Autodesk Inventor part; units mm, degrees
(part 2 of 2)
  line L427 (263.1, -57.6) -> (263.1, -56.8)
  line L428 (263.1, -57.6) -> (263.1, -58.4)
  arc A171 (259.4858, -61.6) -> (260.1929, -61.3071) centre (259.4858, -60.6) ccw
  line L429 (260.1929, -61.3071) -> (263.1, -58.4)
  line L430 (-262.2, 25.9) -> (-263.8, 25.9)
  line L431 (-263.8, 25.9) -> (-267, 22.7)
  line L432 (-267, 22.7) -> (-271.0621, -34.3)
  line L433 (-263.0621, -34.3) -> (-259, 22.7)
  line L434 (-259, 22.7) -> (-262.2, 25.9)
  line L435 (-271.0621, -34.3) -> (-267.8621, -37.5)
  line L436 (-267.8621, -37.5) -> (-266.2621, -37.5)
  line L437 (-266.2621, -37.5) -> (-263.0621, -34.3)
  line L438 (-217, 20.5) -> (-219.9071, 17.5929)
  line L439 (-220.2, 16.8858) -> (-220.2, -0.3)
  line L440 (-237.3858, -0.3) -> (-220.2, -0.3)
  line L441 (-238.0929, -0.5929) -> (-241, -3.5)
  line L442 (-241, -3.5) -> (-241, -5.1)
  line L443 (-237.3858, -8.3) -> (-220.2, -8.3)
  line L444 (-220.2, -8.3) -> (-220.2, -25.4858)
  line L445 (-217, -29.1) -> (-215.4, -29.1)
  line L446 (-215.4, -29.1) -> (-212.4929, -26.1929)
  line L447 (-212.2, -25.4858) -> (-212.2, -8.3)
  line L448 (-195.0142, -0.3) -> (-212.2, -0.3)
  line L449 (-195.0142, -8.3) -> (-212.2, -8.3)
  line L450 (-194.3071, -0.5929) -> (-191.4, -3.5)
  line L451 (-191.4, -3.5) -> (-191.4, -5.1)
  line L452 (-238.0929, -8.0071) -> (-241, -5.1)
  line L453 (-219.9071, -26.1929) -> (-217, -29.1)
  line L454 (-194.3071, -8.0071) -> (-191.4, -5.1)
  line L455 (-212.2, -0.3) -> (-212.2, 16.8858)
  line L456 (-212.4929, 17.5929) -> (-215.4, 20.5)
  line L457 (-215.4, 20.5) -> (-217, 20.5)
  arc A172 (-219.9071, 17.5929) -> (-220.2, 16.8858) centre (-219.2, 16.8858) ccw
  arc A173 (-212.2, 16.8858) -> (-212.4929, 17.5929) centre (-213.2, 16.8858) ccw
  arc A174 (-194.3071, -0.5929) -> (-195.0142, -0.3) centre (-195.0142, -1.3) ccw
  arc A175 (-195.0142, -8.3) -> (-194.3071, -8.0071) centre (-195.0142, -7.3) ccw
  arc A176 (-220.2, -25.4858) -> (-219.9071, -26.1929) centre (-219.2, -25.4858) ccw
  arc A177 (-212.4929, -26.1929) -> (-212.2, -25.4858) centre (-213.2, -25.4858) ccw
  arc A178 (-238.0929, -8.0071) -> (-237.3858, -8.3) centre (-237.3858, -7.3) ccw
  arc A179 (-237.3858, -0.3) -> (-238.0929, -0.5929) centre (-237.3858, -1.3) ccw
  line L458 (-34.2, 15) -> (-32.2, 15)
  line L459 (-32.2, 15) -> (-29, 11.8)
  line L460 (-29, 11.8) -> (-29, 9.8)
  line L461 (-29, 9.8) -> (-32.2, 6.6)
  line L462 (-32.2, 6.6) -> (-34.2, 6.6)
  line L463 (-34.2, 6.6) -> (-37.4, 9.8)
  line L464 (-37.4, 9.8) -> (-37.4, 11.8)
  line L465 (-37.4, 11.8) -> (-34.2, 15)
  line L466 (-34.2, -14.4) -> (-32.2, -14.4)
  line L467 (-32.2, -14.4) -> (-29, -17.6)
  line L468 (-29, -17.6) -> (-29, -19.6)
  line L469 (-29, -19.6) -> (-32.2, -22.8)
  line L470 (-32.2, -22.8) -> (-34.2, -22.8)
  line L471 (-34.2, -22.8) -> (-37.4, -19.6)
  line L472 (-37.4, -19.6) -> (-37.4, -17.6)
  line L473 (-37.4, -17.6) -> (-34.2, -14.4)
  line L474 (121.9, 15) -> (123.9, 15)
  line L475 (123.9, 15) -> (127.1, 11.8)
  line L476 (127.1, 11.8) -> (127.1, 9.8)
  line L477 (127.1, 9.8) -> (123.9, 6.6)
  line L478 (123.9, 6.6) -> (121.9, 6.6)
  line L479 (121.9, 6.6) -> (118.7, 9.8)
  line L480 (118.7, 9.8) -> (118.7, 11.8)
  line L481 (118.7, 11.8) -> (121.9, 15)
  line L482 (121.9, -14.4) -> (123.9, -14.4)
  line L483 (123.9, -14.4) -> (127.1, -17.6)
  line L484 (127.1, -17.6) -> (127.1, -19.6)
  line L485 (127.1, -19.6) -> (123.9, -22.8)
  line L486 (123.9, -22.8) -> (121.9, -22.8)
  line L487 (121.9, -22.8) -> (118.7, -19.6)
  line L488 (118.7, -19.6) -> (118.7, -17.6)
  line L489 (118.7, -17.6) -> (121.9, -14.4)
  point P0 (-22.4267, -1.12)
  dimension "d244" = 0
  dimension "d246" = 0
  dimension "d247" = 0
  dimension "d248" = 0
  dimension "d249" = 10
  dimension "d250" = 7.5
  dimension "d251" = 25
  dimension "d252" = 7.5
  dimension "d253" = 25
  dimension "d308" = 1.1
  dimension "d309" = 21
  dimension "d310" = 21
  dimension "d324" = 21
  dimension "d325" = 0
  dimension "d326" = 21
  dimension "d327" = 21
  dimension "d328" = 0
  dimension "d329" = 21
  dimension "d330" = 39
  dimension "d334" = 0
  dimension "d335" = 18
  dimension "d336" = 23
  dimension "d339" = 11.5
  dimension "d341" = 11.5
sketch "Clock Front Face Outline" plane through (0, 0, 0) normal (0, 0, 1) x (1, 0, 0)
  line L0 (-99.6752, 68) -> (99.6752, 68)
  line L1 (300, 16.6643) -> (300, -28.3498)
  line L2 (-300, -28.3498) -> (-300, 16.6643)
  arc A0 (261.5609, 58.5131) -> (100.3256, 67.9894) centre (0, -3015.4231) ccw
  arc A1 (-100.3256, 67.9894) -> (-261.5609, 58.5131) centre (0, -3015.4231) ccw
  line L3 (-159.5034, -75) -> (159.5034, -75)
  arc A2 (-263.2612, -68.2167) -> (-160.4975, -74.9753) centre (0, 3150) ccw
  arc A3 (160.4975, -74.9753) -> (263.2612, -68.2167) centre (0, 3150) ccw
  arc A4 (300, 16.6643) -> (261.5609, 58.5131) centre (258, 16.6643) ccw
  arc A5 (263.2612, -68.2167) -> (300, -28.3498) centre (260, -28.3498) ccw
  arc A6 (-300, -28.3498) -> (-263.2612, -68.2167) centre (-260, -28.3498) ccw
  arc A7 (-261.5609, 58.5131) -> (-300, 16.6643) centre (-258, 16.6643) ccw
  arc A8 (-99.6752, 68) -> (-100.3256, 67.9894) centre (-99.6752, 48) ccw
  arc A9 (100.3256, 67.9894) -> (99.6752, 68) centre (99.6752, 48) ccw
  arc A10 (159.5034, -75) -> (160.4975, -74.9753) centre (159.5034, -55) ccw
  arc A11 (-160.4975, -74.9753) -> (-159.5034, -75) centre (-159.5034, -55) ccw
  point P0 (0, -2.2582)
  point P1 (-100, 68)
  point P2 (100, 68)
  point P3 (-300, 55)
  point P4 (300, 55)
  point P5 (-300, -65)
  point P6 (300, -65)
  point P7 (-160, -75)
  point P8 (160, -75)
  dimension "d0" = 600
  dimension "d4" = 120
  dimension "d5" = 120
  dimension "d12" = 140
  dimension "d13" = 140
  dimension "d14" = 200
  dimension "d15" = 200
  dimension "d16" = 200
  dimension "d17" = 320
  dimension "d18" = 143
  dimension "d19" = 10
  dimension "d20" = 10
  dimension "d21" = 13
  dimension "d22" = 13
  dimension "d24" = 42
  dimension "d25" = 40
  dimension "d26" = 40
  dimension "d27" = 42
  dimension "d28" = 20
  measures "d0" distance between parallel lines of L1 L2
  measures "d4" distance of point (-300, 55) point (-300, -65)
  measures "d5" distance of point (300, 55) point (300, -65)
  measures "d12" horizontal distance of point (-300, -65) point (-160, -75)
  measures "d13" horizontal distance of point (300, -65) point (160, -75)
  measures "d14" horizontal distance of point (-300, 55) point (-100, 68)
  measures "d15" horizontal distance of point (300, 55) point (100, 68)
  measures "d16" distance of point (100, 68) point (-100, 68)
  measures "d17" distance of point (160, -75) point (-160, -75)
  measures "d18" distance from line of L3 point (-100, 68)
  measures "d19" vertical distance of point (-300, -65) point (-160, -75)
  measures "d20" vertical distance of point (300, -65) point (160, -75)
  measures "d21" vertical distance of point (100, 68) point (300, 55)
  measures "d22" vertical distance of point (-100, 68) point (-300, 55)
  measures "d24" radius of A4
  measures "d25" radius of A5
  measures "d26" radius of A6
  measures "d27" radius of A7
  measures "d28" radius of A8
sketch "Sketch1" plane through (0, 0, 0) normal (0, 0, 1) x (1, 0, 0)
  line L0 (-99.6752, 68) -> (99.6752, 68)
  line L1 (300, 16.6643) -> (300, -28.3498)
  line L2 (-300, -28.3498) -> (-300, 16.6643)
  arc A0 (261.5609, 58.5131) -> (100.3256, 67.9894) centre (0, -3015.4231) ccw
  arc A1 (-100.3256, 67.9894) -> (-261.5609, 58.5131) centre (0, -3015.4231) ccw
  line L3 (-159.5034, -75) -> (159.5034, -75)
  arc A2 (-263.2612, -68.2167) -> (-160.4975, -74.9753) centre (0, 3150) ccw
  arc A3 (160.4975, -74.9753) -> (263.2612, -68.2167) centre (0, 3150) ccw
  arc A4 (300, 16.6643) -> (261.5609, 58.5131) centre (258, 16.6643) ccw
  arc A5 (263.2612, -68.2167) -> (300, -28.3498) centre (260, -28.3498) ccw
  arc A6 (-300, -28.3498) -> (-263.2612, -68.2167) centre (-260, -28.3498) ccw
  arc A7 (-261.5609, 58.5131) -> (-300, 16.6643) centre (-258, 16.6643) ccw
  arc A8 (-99.6752, 68) -> (-100.3256, 67.9894) centre (-99.6752, 48) ccw
  arc A9 (100.3256, 67.9894) -> (99.6752, 68) centre (99.6752, 48) ccw
  arc A10 (159.5034, -75) -> (160.4975, -74.9753) centre (159.5034, -55) ccw
  arc A11 (-160.4975, -74.9753) -> (-159.5034, -75) centre (-159.5034, -55) ccw
  point P0 (0, 0)
  dimension "d2" = 300
  dimension "d23" = 75
extrude "Extrusion1" add sketch "Sketch1" along normal blind 3
sketch "Sketch4" plane through (0, 0, 3) normal (0, 0, 1) x (1, 0, 0)
  line L0 (-300, 16.6643) -> (-300, -28.3498) projected
  line L1 (99.6752, 68) -> (-99.6752, 68) projected
  line L2 (-159.5034, -75) -> (159.5034, -75) projected
  line L3 (300, -28.3498) -> (300, 16.6643) projected
  arc A0 (144.2071, 46.2929) -> (144.9142, 46) centre (144.9142, 47) ccw
  arc A1 (144.9142, 54) -> (144.2071, 53.7071) centre (144.9142, 53) ccw
  line L4 (144.2071, 46.2929) -> (141.3, 49.2)
  line L5 (144.2071, 53.7071) -> (141.3, 50.8)
  line L6 (141.3, 50) -> (141.3, 49.2)
  line L7 (141.3, 50) -> (141.3, 50.8)
  line L8 (144.9142, 54) -> (187.6858, 54)
  line L9 (187.6858, 46) -> (144.9142, 46)
  arc A2 (188.3929, 53.7071) -> (187.6858, 54) centre (187.6858, 53) ccw
  line L10 (188.3929, 53.7071) -> (191.3, 50.8)
  line L11 (191.3, 50) -> (191.3, 50.8)
  line L12 (191.3, 50) -> (191.3, 49.2)
  arc A3 (187.6858, 46) -> (188.3929, 46.2929) centre (187.6858, 47) ccw
  line L13 (188.3929, 46.2929) -> (191.3, 49.2)
  arc A4 (144.2071, -7.5071) -> (144.9142, -7.8) centre (144.9142, -6.8) ccw
  arc A5 (144.9142, 0.2) -> (144.2071, -0.0929) centre (144.9142, -0.8) ccw
  line L14 (144.2071, -7.5071) -> (141.3, -4.6)
  line L15 (144.2071, -0.0929) -> (141.3, -3)
  line L16 (141.3, -3.8) -> (141.3, -4.6)
  line L17 (141.3, -3.8) -> (141.3, -3)
  line L18 (144.9142, 0.2) -> (187.6858, 0.2)
  line L19 (187.6858, -7.8) -> (144.9142, -7.8)
  arc A6 (188.3929, -0.0929) -> (187.6858, 0.2) centre (187.6858, -0.8) ccw
  line L20 (188.3929, -0.0929) -> (191.3, -3)
  line L21 (191.3, -3.8) -> (191.3, -3)
  line L22 (191.3, -3.8) -> (191.3, -4.6)
  arc A7 (187.6858, -7.8) -> (188.3929, -7.5071) centre (187.6858, -6.8) ccw
  line L23 (188.3929, -7.5071) -> (191.3, -4.6)
  arc A8 (143.1071, 1.0071) -> (143.4, 1.7142) centre (142.4, 1.7142) ccw
  arc A9 (135.4, 1.7142) -> (135.6929, 1.0071) centre (136.4, 1.7142) ccw
  line L24 (143.1071, 1.0071) -> (140.2, -1.9)
  line L25 (135.6929, 1.0071) -> (138.6, -1.9)
  line L26 (139.4, -1.9) -> (140.2, -1.9)
  line L27 (139.4, -1.9) -> (138.6, -1.9)
  line L28 (135.4, 1.7142) -> (135.4, 44.4858)
  line L29 (143.4, 44.4858) -> (143.4, 1.7142)
  arc A10 (135.6929, 45.1929) -> (135.4, 44.4858) centre (136.4, 44.4858) ccw
  line L30 (135.6929, 45.1929) -> (138.6, 48.1)
  line L31 (139.4, 48.1) -> (138.6, 48.1)
  line L32 (139.4, 48.1) -> (140.2, 48.1)
  arc A11 (143.4, 44.4858) -> (143.1071, 45.1929) centre (142.4, 44.4858) ccw
  line L33 (143.1071, 45.1929) -> (140.2, 48.1)
  arc A12 (143.1071, -52.7929) -> (143.4, -52.0858) centre (142.4, -52.0858) ccw
  arc A13 (135.4, -52.0858) -> (135.6929, -52.7929) centre (136.4, -52.0858) ccw
  line L34 (143.1071, -52.7929) -> (140.2, -55.7)
  line L35 (135.6929, -52.7929) -> (138.6, -55.7)
  line L36 (139.4, -55.7) -> (140.2, -55.7)
  line L37 (139.4, -55.7) -> (138.6, -55.7)
  line L38 (135.4, -52.0858) -> (135.4, -9.3142)
  line L39 (143.4, -9.3142) -> (143.4, -52.0858)
  arc A14 (135.6929, -8.6071) -> (135.4, -9.3142) centre (136.4, -9.3142) ccw
  line L40 (135.6929, -8.6071) -> (138.6, -5.7)
  line L41 (139.4, -5.7) -> (138.6, -5.7)
  line L42 (139.4, -5.7) -> (140.2, -5.7)
  arc A15 (143.4, -9.3142) -> (143.1071, -8.6071) centre (142.4, -9.3142) ccw
  line L43 (143.1071, -8.6071) -> (140.2, -5.7)
  arc A16 (196.9071, 1.0071) -> (197.2, 1.7142) centre (196.2, 1.7142) ccw
  arc A17 (189.2, 1.7142) -> (189.4929, 1.0071) centre (190.2, 1.7142) ccw
  line L44 (196.9071, 1.0071) -> (194, -1.9)
  line L45 (189.4929, 1.0071) -> (192.4, -1.9)
  line L46 (193.2, -1.9) -> (194, -1.9)
  line L47 (193.2, -1.9) -> (192.4, -1.9)
  line L48 (189.2, 1.7142) -> (189.2, 44.4858)
  line L49 (197.2, 44.4858) -> (197.2, 1.7142)
  arc A18 (189.4929, 45.1929) -> (189.2, 44.4858) centre (190.2, 44.4858) ccw
  line L50 (189.4929, 45.1929) -> (192.4, 48.1)
  line L51 (193.2, 48.1) -> (192.4, 48.1)
  line L52 (193.2, 48.1) -> (194, 48.1)
  arc A19 (197.2, 44.4858) -> (196.9071, 45.1929) centre (196.2, 44.4858) ccw
  line L53 (196.9071, 45.1929) -> (194, 48.1)
  arc A20 (196.9071, -52.7929) -> (197.2, -52.0858) centre (196.2, -52.0858) ccw
  arc A21 (189.2, -52.0858) -> (189.4929, -52.7929) centre (190.2, -52.0858) ccw
  line L54 (196.9071, -52.7929) -> (194, -55.7)
  line L55 (189.4929, -52.7929) -> (192.4, -55.7)
  line L56 (193.2, -55.7) -> (194, -55.7)
  line L57 (193.2, -55.7) -> (192.4, -55.7)
  line L58 (189.2, -52.0858) -> (189.2, -9.3142)
  line L59 (197.2, -9.3142) -> (197.2, -52.0858)
  arc A22 (189.4929, -8.6071) -> (189.2, -9.3142) centre (190.2, -9.3142) ccw
  line L60 (189.4929, -8.6071) -> (192.4, -5.7)
  line L61 (193.2, -5.7) -> (192.4, -5.7)
  line L62 (193.2, -5.7) -> (194, -5.7)
  arc A23 (197.2, -9.3142) -> (196.9071, -8.6071) centre (196.2, -9.3142) ccw
  line L63 (196.9071, -8.6071) -> (194, -5.7)
  arc A24 (144.2071, -61.3071) -> (144.9142, -61.6) centre (144.9142, -60.6) ccw
  arc A25 (144.9142, -53.6) -> (144.2071, -53.8929) centre (144.9142, -54.6) ccw
  line L64 (144.2071, -61.3071) -> (141.3, -58.4)
  line L65 (144.2071, -53.8929) -> (141.3, -56.8)
  line L66 (141.3, -57.6) -> (141.3, -58.4)
  line L67 (141.3, -57.6) -> (141.3, -56.8)
  line L68 (144.9142, -53.6) -> (187.6858, -53.6)
  line L69 (187.6858, -61.6) -> (144.9142, -61.6)
  arc A26 (188.3929, -53.8929) -> (187.6858, -53.6) centre (187.6858, -54.6) ccw
  line L70 (188.3929, -53.8929) -> (191.3, -56.8)
  line L71 (191.3, -57.6) -> (191.3, -56.8)
  line L72 (191.3, -57.6) -> (191.3, -58.4)
  arc A27 (187.6858, -61.6) -> (188.3929, -61.3071) centre (187.6858, -60.6) ccw
  line L73 (188.3929, -61.3071) -> (191.3, -58.4)
  arc A28 (57.4071, 46.2929) -> (58.1142, 46) centre (58.1142, 47) ccw
  arc A29 (58.1142, 54) -> (57.4071, 53.7071) centre (58.1142, 53) ccw
  line L74 (57.4071, 46.2929) -> (54.5, 49.2)
  line L75 (57.4071, 53.7071) -> (54.5, 50.8)
  line L76 (54.5, 50) -> (54.5, 49.2)
  line L77 (54.5, 50) -> (54.5, 50.8)
  line L78 (58.1142, 54) -> (100.8858, 54)
  line L79 (100.8858, 46) -> (58.1142, 46)
  arc A30 (101.5929, 53.7071) -> (100.8858, 54) centre (100.8858, 53) ccw
  line L80 (101.5929, 53.7071) -> (104.5, 50.8)
  line L81 (104.5, 50) -> (104.5, 50.8)
  line L82 (104.5, 50) -> (104.5, 49.2)
  arc A31 (100.8858, 46) -> (101.5929, 46.2929) centre (100.8858, 47) ccw
  line L83 (101.5929, 46.2929) -> (104.5, 49.2)
  arc A32 (57.4071, -7.5071) -> (58.1142, -7.8) centre (58.1142, -6.8) ccw
  arc A33 (58.1142, 0.2) -> (57.4071, -0.0929) centre (58.1142, -0.8) ccw
  line L84 (57.4071, -7.5071) -> (54.5, -4.6)
  line L85 (57.4071, -0.0929) -> (54.5, -3)
  line L86 (54.5, -3.8) -> (54.5, -4.6)
  line L87 (54.5, -3.8) -> (54.5, -3)
  line L88 (58.1142, 0.2) -> (100.8858, 0.2)
  line L89 (100.8858, -7.8) -> (58.1142, -7.8)
  arc A34 (101.5929, -0.0929) -> (100.8858, 0.2) centre (100.8858, -0.8) ccw
  line L90 (101.5929, -0.0929) -> (104.5, -3)
  line L91 (104.5, -3.8) -> (104.5, -3)
  line L92 (104.5, -3.8) -> (104.5, -4.6)
  arc A35 (100.8858, -7.8) -> (101.5929, -7.5071) centre (100.8858, -6.8) ccw
  line L93 (101.5929, -7.5071) -> (104.5, -4.6)
  arc A36 (56.3071, 1.0071) -> (56.6, 1.7142) centre (55.6, 1.7142) ccw
  arc A37 (48.6, 1.7142) -> (48.8929, 1.0071) centre (49.6, 1.7142) ccw
  line L94 (56.3071, 1.0071) -> (53.4, -1.9)
  line L95 (48.8929, 1.0071) -> (51.8, -1.9)
  line L96 (52.6, -1.9) -> (53.4, -1.9)
  line L97 (52.6, -1.9) -> (51.8, -1.9)
  line L98 (48.6, 1.7142) -> (48.6, 44.4858)
  line L99 (56.6, 44.4858) -> (56.6, 1.7142)
  arc A38 (48.8929, 45.1929) -> (48.6, 44.4858) centre (49.6, 44.4858) ccw
  line L100 (48.8929, 45.1929) -> (51.8, 48.1)
  line L101 (52.6, 48.1) -> (51.8, 48.1)
  line L102 (52.6, 48.1) -> (53.4, 48.1)
  arc A39 (56.6, 44.4858) -> (56.3071, 45.1929) centre (55.6, 44.4858) ccw
  line L103 (56.3071, 45.1929) -> (53.4, 48.1)
  arc A40 (56.3071, -52.7929) -> (56.6, -52.0858) centre (55.6, -52.0858) ccw
  arc A41 (48.6, -52.0858) -> (48.8929, -52.7929) centre (49.6, -52.0858) ccw
  line L104 (56.3071, -52.7929) -> (53.4, -55.7)
  line L105 (48.8929, -52.7929) -> (51.8, -55.7)
  line L106 (52.6, -55.7) -> (53.4, -55.7)
  line L107 (52.6, -55.7) -> (51.8, -55.7)
  line L108 (48.6, -52.0858) -> (48.6, -9.3142)
  line L109 (56.6, -9.3142) -> (56.6, -52.0858)
  arc A42 (48.8929, -8.6071) -> (48.6, -9.3142) centre (49.6, -9.3142) ccw
  line L110 (48.8929, -8.6071) -> (51.8, -5.7)
  line L111 (52.6, -5.7) -> (51.8, -5.7)
  line L112 (52.6, -5.7) -> (53.4, -5.7)
  arc A43 (56.6, -9.3142) -> (56.3071, -8.6071) centre (55.6, -9.3142) ccw
  line L113 (56.3071, -8.6071) -> (53.4, -5.7)
  arc A44 (110.1071, 1.0071) -> (110.4, 1.7142) centre (109.4, 1.7142) ccw
  arc A45 (102.4, 1.7142) -> (102.6929, 1.0071) centre (103.4, 1.7142) ccw
  line L114 (110.1071, 1.0071) -> (107.2, -1.9)
  line L115 (102.6929, 1.0071) -> (105.6, -1.9)
  line L116 (106.4, -1.9) -> (107.2, -1.9)
  line L117 (106.4, -1.9) -> (105.6, -1.9)
  line L118 (102.4, 1.7142) -> (102.4, 44.4858)
  line L119 (110.4, 44.4858) -> (110.4, 1.7142)
  arc A46 (102.6929, 45.1929) -> (102.4, 44.4858) centre (103.4, 44.4858) ccw
  line L120 (102.6929, 45.1929) -> (105.6, 48.1)
  line L121 (106.4, 48.1) -> (105.6, 48.1)
  line L122 (106.4, 48.1) -> (107.2, 48.1)
  arc A47 (110.4, 44.4858) -> (110.1071, 45.1929) centre (109.4, 44.4858) ccw
  line L123 (110.1071, 45.1929) -> (107.2, 48.1)
  arc A48 (110.1071, -52.7929) -> (110.4, -52.0858) centre (109.4, -52.0858) ccw
  arc A49 (102.4, -52.0858) -> (102.6929, -52.7929) centre (103.4, -52.0858) ccw
  line L124 (110.1071, -52.7929) -> (107.2, -55.7)
  line L125 (102.6929, -52.7929) -> (105.6, -55.7)
  line L126 (106.4, -55.7) -> (107.2, -55.7)
  line L127 (106.4, -55.7) -> (105.6, -55.7)
  line L128 (102.4, -52.0858) -> (102.4, -9.3142)
  line L129 (110.4, -9.3142) -> (110.4, -52.0858)
  arc A50 (102.6929, -8.6071) -> (102.4, -9.3142) centre (103.4, -9.3142) ccw
  line L130 (102.6929, -8.6071) -> (105.6, -5.7)
  line L131 (106.4, -5.7) -> (105.6, -5.7)
  line L132 (106.4, -5.7) -> (107.2, -5.7)
  arc A51 (110.4, -9.3142) -> (110.1071, -8.6071) centre (109.4, -9.3142) ccw
  line L133 (110.1071, -8.6071) -> (107.2, -5.7)
  arc A52 (57.4071, -61.3071) -> (58.1142, -61.6) centre (58.1142, -60.6) ccw
  arc A53 (58.1142, -53.6) -> (57.4071, -53.8929) centre (58.1142, -54.6) ccw
  line L134 (57.4071, -61.3071) -> (54.5, -58.4)
  line L135 (57.4071, -53.8929) -> (54.5, -56.8)
  line L136 (54.5, -57.6) -> (54.5, -58.4)
  line L137 (54.5, -57.6) -> (54.5, -56.8)
  line L138 (58.1142, -53.6) -> (100.8858, -53.6)
  line L139 (100.8858, -61.6) -> (58.1142, -61.6)
  arc A54 (101.5929, -53.8929) -> (100.8858, -53.6) centre (100.8858, -54.6) ccw
  line L140 (101.5929, -53.8929) -> (104.5, -56.8)
  line L141 (104.5, -57.6) -> (104.5, -56.8)
  line L142 (104.5, -57.6) -> (104.5, -58.4)
  arc A55 (100.8858, -61.6) -> (101.5929, -61.3071) centre (100.8858, -60.6) ccw
  line L143 (101.5929, -61.3071) -> (104.5, -58.4)
  arc A56 (-11.8929, 46.2929) -> (-11.1858, 46) centre (-11.1858, 47) ccw
  arc A57 (-11.1858, 54) -> (-11.8929, 53.7071) centre (-11.1858, 53) ccw
  line L144 (-11.8929, 46.2929) -> (-14.8, 49.2)
  line L145 (-11.8929, 53.7071) -> (-14.8, 50.8)
  line L146 (-14.8, 50) -> (-14.8, 49.2)
  line L147 (-14.8, 50) -> (-14.8, 50.8)
  line L148 (-11.1858, 54) -> (31.5858, 54)
  line L149 (31.5858, 46) -> (-11.1858, 46)
  arc A58 (32.2929, 53.7071) -> (31.5858, 54) centre (31.5858, 53) ccw
  line L150 (32.2929, 53.7071) -> (35.2, 50.8)
  line L151 (35.2, 50) -> (35.2, 50.8)
  line L152 (35.2, 50) -> (35.2, 49.2)
  arc A59 (31.5858, 46) -> (32.2929, 46.2929) centre (31.5858, 47) ccw
  line L153 (32.2929, 46.2929) -> (35.2, 49.2)
  arc A60 (-11.8929, -7.5071) -> (-11.1858, -7.8) centre (-11.1858, -6.8) ccw
  arc A61 (-11.1858, 0.2) -> (-11.8929, -0.0929) centre (-11.1858, -0.8) ccw
  line L154 (-11.8929, -7.5071) -> (-14.8, -4.6)
  line L155 (-11.8929, -0.0929) -> (-14.8, -3)
  line L156 (-14.8, -3.8) -> (-14.8, -4.6)
  line L157 (-14.8, -3.8) -> (-14.8, -3)
  line L158 (-11.1858, 0.2) -> (31.5858, 0.2)
  line L159 (31.5858, -7.8) -> (-11.1858, -7.8)
  arc A62 (32.2929, -0.0929) -> (31.5858, 0.2) centre (31.5858, -0.8) ccw
  line L160 (32.2929, -0.0929) -> (35.2, -3)
  line L161 (35.2, -3.8) -> (35.2, -3)
  line L162 (35.2, -3.8) -> (35.2, -4.6)
  arc A63 (31.5858, -7.8) -> (32.2929, -7.5071) centre (31.5858, -6.8) ccw
  line L163 (32.2929, -7.5071) -> (35.2, -4.6)
  arc A64 (-12.9929, 1.0071) -> (-12.7, 1.7142) centre (-13.7, 1.7142) ccw
  arc A65 (-20.7, 1.7142) -> (-20.4071, 1.0071) centre (-19.7, 1.7142) ccw
  line L164 (-12.9929, 1.0071) -> (-15.9, -1.9)
  line L165 (-20.4071, 1.0071) -> (-17.5, -1.9)
  line L166 (-16.7, -1.9) -> (-15.9, -1.9)
  line L167 (-16.7, -1.9) -> (-17.5, -1.9)
  line L168 (-20.7, 1.7142) -> (-20.7, 44.4858)
  line L169 (-12.7, 44.4858) -> (-12.7, 1.7142)
  arc A66 (-20.4071, 45.1929) -> (-20.7, 44.4858) centre (-19.7, 44.4858) ccw
  line L170 (-20.4071, 45.1929) -> (-17.5, 48.1)
  line L171 (-16.7, 48.1) -> (-17.5, 48.1)
  line L172 (-16.7, 48.1) -> (-15.9, 48.1)
  arc A67 (-12.7, 44.4858) -> (-12.9929, 45.1929) centre (-13.7, 44.4858) ccw
  line L173 (-12.9929, 45.1929) -> (-15.9, 48.1)
  arc A68 (-12.9929, -52.7929) -> (-12.7, -52.0858) centre (-13.7, -52.0858) ccw
  arc A69 (-20.7, -52.0858) -> (-20.4071, -52.7929) centre (-19.7, -52.0858) ccw
  line L174 (-12.9929, -52.7929) -> (-15.9, -55.7)
  line L175 (-20.4071, -52.7929) -> (-17.5, -55.7)
  line L176 (-16.7, -55.7) -> (-15.9, -55.7)
  line L177 (-16.7, -55.7) -> (-17.5, -55.7)
  line L178 (-20.7, -52.0858) -> (-20.7, -9.3142)
  line L179 (-12.7, -9.3142) -> (-12.7, -52.0858)
  arc A70 (-20.4071, -8.6071) -> (-20.7, -9.3142) centre (-19.7, -9.3142) ccw
  line L180 (-20.4071, -8.6071) -> (-17.5, -5.7)
  line L181 (-16.7, -5.7) -> (-17.5, -5.7)
  line L182 (-16.7, -5.7) -> (-15.9, -5.7)
  arc A71 (-12.7, -9.3142) -> (-12.9929, -8.6071) centre (-13.7, -9.3142) ccw
  line L183 (-12.9929, -8.6071) -> (-15.9, -5.7)
  arc A72 (40.8071, 1.0071) -> (41.1, 1.7142) centre (40.1, 1.7142) ccw
  arc A73 (33.1, 1.7142) -> (33.3929, 1.0071) centre (34.1, 1.7142) ccw
  line L184 (40.8071, 1.0071) -> (37.9, -1.9)
  line L185 (33.3929, 1.0071) -> (36.3, -1.9)
  line L186 (37.1, -1.9) -> (37.9, -1.9)
  line L187 (37.1, -1.9) -> (36.3, -1.9)
  line L188 (33.1, 1.7142) -> (33.1, 44.4858)
  line L189 (41.1, 44.4858) -> (41.1, 1.7142)
  arc A74 (33.3929, 45.1929) -> (33.1, 44.4858) centre (34.1, 44.4858) ccw
  line L190 (33.3929, 45.1929) -> (36.3, 48.1)
  line L191 (37.1, 48.1) -> (36.3, 48.1)
  line L192 (37.1, 48.1) -> (37.9, 48.1)
  arc A75 (41.1, 44.4858) -> (40.8071, 45.1929) centre (40.1, 44.4858) ccw
  line L193 (40.8071, 45.1929) -> (37.9, 48.1)
  arc A76 (40.8071, -52.7929) -> (41.1, -52.0858) centre (40.1, -52.0858) ccw
  arc A77 (33.1, -52.0858) -> (33.3929, -52.7929) centre (34.1, -52.0858) ccw
  line L194 (40.8071, -52.7929) -> (37.9, -55.7)
  line L195 (33.3929, -52.7929) -> (36.3, -55.7)
  line L196 (37.1, -55.7) -> (37.9, -55.7)
  line L197 (37.1, -55.7) -> (36.3, -55.7)
  line L198 (33.1, -52.0858) -> (33.1, -9.3142)
  line L199 (41.1, -9.3142) -> (41.1, -52.0858)
  arc A78 (33.3929, -8.6071) -> (33.1, -9.3142) centre (34.1, -9.3142) ccw
  line L200 (33.3929, -8.6071) -> (36.3, -5.7)
  line L201 (37.1, -5.7) -> (36.3, -5.7)
  line L202 (37.1, -5.7) -> (37.9, -5.7)
  arc A79 (41.1, -9.3142) -> (40.8071, -8.6071) centre (40.1, -9.3142) ccw
  line L203 (40.8071, -8.6071) -> (37.9, -5.7)
  arc A80 (-11.8929, -61.3071) -> (-11.1858, -61.6) centre (-11.1858, -60.6) ccw
  arc A81 (-11.1858, -53.6) -> (-11.8929, -53.8929) centre (-11.1858, -54.6) ccw
  line L204 (-11.8929, -61.3071) -> (-14.8, -58.4)
  line L205 (-11.8929, -53.8929) -> (-14.8, -56.8)
  line L206 (-14.8, -57.6) -> (-14.8, -58.4)
  line L207 (-14.8, -57.6) -> (-14.8, -56.8)
  line L208 (-11.1858, -53.6) -> (31.5858, -53.6)
  line L209 (31.5858, -61.6) -> (-11.1858, -61.6)
  arc A82 (32.2929, -53.8929) -> (31.5858, -53.6) centre (31.5858, -54.6) ccw
  line L210 (32.2929, -53.8929) -> (35.2, -56.8)
  line L211 (35.2, -57.6) -> (35.2, -56.8)
  line L212 (35.2, -57.6) -> (35.2, -58.4)
  arc A83 (31.5858, -61.6) -> (32.2929, -61.3071) centre (31.5858, -60.6) ccw
  line L213 (32.2929, -61.3071) -> (35.2, -58.4)
  arc A84 (-98.6929, 46.2929) -> (-97.9858, 46) centre (-97.9858, 47) ccw
  arc A85 (-97.9858, 54) -> (-98.6929, 53.7071) centre (-97.9858, 53) ccw
  line L214 (-98.6929, 46.2929) -> (-101.6, 49.2)
  line L215 (-98.6929, 53.7071) -> (-101.6, 50.8)
  line L216 (-101.6, 50) -> (-101.6, 49.2)
  line L217 (-101.6, 50) -> (-101.6, 50.8)
  line L218 (-97.9858, 54) -> (-55.2142, 54)
  line L219 (-55.2142, 46) -> (-97.9858, 46)
  arc A86 (-54.5071, 53.7071) -> (-55.2142, 54) centre (-55.2142, 53) ccw
  line L220 (-54.5071, 53.7071) -> (-51.6, 50.8)
  line L221 (-51.6, 50) -> (-51.6, 50.8)
  line L222 (-51.6, 50) -> (-51.6, 49.2)
  arc A87 (-55.2142, 46) -> (-54.5071, 46.2929) centre (-55.2142, 47) ccw
  line L223 (-54.5071, 46.2929) -> (-51.6, 49.2)
  arc A88 (-98.6929, -7.5071) -> (-97.9858, -7.8) centre (-97.9858, -6.8) ccw
  arc A89 (-97.9858, 0.2) -> (-98.6929, -0.0929) centre (-97.9858, -0.8) ccw
  line L224 (-98.6929, -7.5071) -> (-101.6, -4.6)
  line L225 (-98.6929, -0.0929) -> (-101.6, -3)
  line L226 (-101.6, -3.8) -> (-101.6, -4.6)
  line L227 (-101.6, -3.8) -> (-101.6, -3)
  line L228 (-97.9858, 0.2) -> (-55.2142, 0.2)
  line L229 (-55.2142, -7.8) -> (-97.9858, -7.8)
  arc A90 (-54.5071, -0.0929) -> (-55.2142, 0.2) centre (-55.2142, -0.8) ccw
  line L230 (-54.5071, -0.0929) -> (-51.6, -3)
  line L231 (-51.6, -3.8) -> (-51.6, -3)
  line L232 (-51.6, -3.8) -> (-51.6, -4.6)
  arc A91 (-55.2142, -7.8) -> (-54.5071, -7.5071) centre (-55.2142, -6.8) ccw
  line L233 (-54.5071, -7.5071) -> (-51.6, -4.6)
  arc A92 (-99.7929, 1.0071) -> (-99.5, 1.7142) centre (-100.5, 1.7142) ccw
  arc A93 (-107.5, 1.7142) -> (-107.2071, 1.0071) centre (-106.5, 1.7142) ccw
  line L234 (-99.7929, 1.0071) -> (-102.7, -1.9)
  line L235 (-107.2071, 1.0071) -> (-104.3, -1.9)
  line L236 (-103.5, -1.9) -> (-102.7, -1.9)
  line L237 (-103.5, -1.9) -> (-104.3, -1.9)
  line L238 (-107.5, 1.7142) -> (-107.5, 44.4858)
  line L239 (-99.5, 44.4858) -> (-99.5, 1.7142)
  arc A94 (-107.2071, 45.1929) -> (-107.5, 44.4858) centre (-106.5, 44.4858) ccw
  line L240 (-107.2071, 45.1929) -> (-104.3, 48.1)
  line L241 (-103.5, 48.1) -> (-104.3, 48.1)
  line L242 (-103.5, 48.1) -> (-102.7, 48.1)
  arc A95 (-99.5, 44.4858) -> (-99.7929, 45.1929) centre (-100.5, 44.4858) ccw
  line L243 (-99.7929, 45.1929) -> (-102.7, 48.1)
  arc A96 (-99.7929, -52.7929) -> (-99.5, -52.0858) centre (-100.5, -52.0858) ccw
  arc A97 (-107.5, -52.0858) -> (-107.2071, -52.7929) centre (-106.5, -52.0858) ccw
  line L244 (-99.7929, -52.7929) -> (-102.7, -55.7)
  line L245 (-107.2071, -52.7929) -> (-104.3, -55.7)
  line L246 (-103.5, -55.7) -> (-102.7, -55.7)
  line L247 (-103.5, -55.7) -> (-104.3, -55.7)
  line L248 (-107.5, -52.0858) -> (-107.5, -9.3142)
  line L249 (-99.5, -9.3142) -> (-99.5, -52.0858)
  arc A98 (-107.2071, -8.6071) -> (-107.5, -9.3142) centre (-106.5, -9.3142) ccw
  line L250 (-107.2071, -8.6071) -> (-104.3, -5.7)
  line L251 (-103.5, -5.7) -> (-104.3, -5.7)
  line L252 (-103.5, -5.7) -> (-102.7, -5.7)
  arc A99 (-99.5, -9.3142) -> (-99.7929, -8.6071) centre (-100.5, -9.3142) ccw
  line L253 (-99.7929, -8.6071) -> (-102.7, -5.7)
  arc A100 (-45.9929, 1.0071) -> (-45.7, 1.7142) centre (-46.7, 1.7142) ccw
  arc A101 (-53.7, 1.7142) -> (-53.4071, 1.0071) centre (-52.7, 1.7142) ccw
  line L254 (-45.9929, 1.0071) -> (-48.9, -1.9)
  line L255 (-53.4071, 1.0071) -> (-50.5, -1.9)
  line L256 (-49.7, -1.9) -> (-48.9, -1.9)
  line L257 (-49.7, -1.9) -> (-50.5, -1.9)
  line L258 (-53.7, 1.7142) -> (-53.7, 44.4858)
  line L259 (-45.7, 44.4858) -> (-45.7, 1.7142)
  arc A102 (-53.4071, 45.1929) -> (-53.7, 44.4858) centre (-52.7, 44.4858) ccw
  line L260 (-53.4071, 45.1929) -> (-50.5, 48.1)
  line L261 (-49.7, 48.1) -> (-50.5, 48.1)
  line L262 (-49.7, 48.1) -> (-48.9, 48.1)
  arc A103 (-45.7, 44.4858) -> (-45.9929, 45.1929) centre (-46.7, 44.4858) ccw
  line L263 (-45.9929, 45.1929) -> (-48.9, 48.1)
  arc A104 (-45.9929, -52.7929) -> (-45.7, -52.0858) centre (-46.7, -52.0858) ccw
  arc A105 (-53.7, -52.0858) -> (-53.4071, -52.7929) centre (-52.7, -52.0858) ccw
  line L264 (-45.9929, -52.7929) -> (-48.9, -55.7)
  line L265 (-53.4071, -52.7929) -> (-50.5, -55.7)
  line L266 (-49.7, -55.7) -> (-48.9, -55.7)
  line L267 (-49.7, -55.7) -> (-50.5, -55.7)
  line L268 (-53.7, -52.0858) -> (-53.7, -9.3142)
  line L269 (-45.7, -9.3142) -> (-45.7, -52.0858)
  arc A106 (-53.4071, -8.6071) -> (-53.7, -9.3142) centre (-52.7, -9.3142) ccw
  line L270 (-53.4071, -8.6071) -> (-50.5, -5.7)
  line L271 (-49.7, -5.7) -> (-50.5, -5.7)
  line L272 (-49.7, -5.7) -> (-48.9, -5.7)
  arc A107 (-45.7, -9.3142) -> (-45.9929, -8.6071) centre (-46.7, -9.3142) ccw
  line L273 (-45.9929, -8.6071) -> (-48.9, -5.7)
  arc A108 (-98.6929, -61.3071) -> (-97.9858, -61.6) centre (-97.9858, -60.6) ccw
  arc A109 (-97.9858, -53.6) -> (-98.6929, -53.8929) centre (-97.9858, -54.6) ccw
  line L274 (-98.6929, -61.3071) -> (-101.6, -58.4)
  line L275 (-98.6929, -53.8929) -> (-101.6, -56.8)
  line L276 (-101.6, -57.6) -> (-101.6, -58.4)
  line L277 (-101.6, -57.6) -> (-101.6, -56.8)
  line L278 (-97.9858, -53.6) -> (-55.2142, -53.6)
  line L279 (-55.2142, -61.6) -> (-97.9858, -61.6)
  arc A110 (-54.5071, -53.8929) -> (-55.2142, -53.6) centre (-55.2142, -54.6) ccw
  line L280 (-54.5071, -53.8929) -> (-51.6, -56.8)
  line L281 (-51.6, -57.6) -> (-51.6, -56.8)
  line L282 (-51.6, -57.6) -> (-51.6, -58.4)
  arc A111 (-55.2142, -61.6) -> (-54.5071, -61.3071) centre (-55.2142, -60.6) ccw
  line L283 (-54.5071, -61.3071) -> (-51.6, -58.4)
  arc A112 (-167.9929, 46.2929) -> (-167.2858, 46) centre (-167.2858, 47) ccw
  arc A113 (-167.2858, 54) -> (-167.9929, 53.7071) centre (-167.2858, 53) ccw
  line L284 (-167.9929, 46.2929) -> (-170.9, 49.2)
  line L285 (-167.9929, 53.7071) -> (-170.9, 50.8)
  line L286 (-170.9, 50) -> (-170.9, 49.2)
  line L287 (-170.9, 50) -> (-170.9, 50.8)
  line L288 (-167.2858, 54) -> (-124.5142, 54)
  line L289 (-124.5142, 46) -> (-167.2858, 46)
  arc A114 (-123.8071, 53.7071) -> (-124.5142, 54) centre (-124.5142, 53) ccw
  line L290 (-123.8071, 53.7071) -> (-120.9, 50.8)
  line L291 (-120.9, 50) -> (-120.9, 50.8)
  line L292 (-120.9, 50) -> (-120.9, 49.2)
  arc A115 (-124.5142, 46) -> (-123.8071, 46.2929) centre (-124.5142, 47) ccw
  line L293 (-123.8071, 46.2929) -> (-120.9, 49.2)
  arc A116 (-167.9929, -7.5071) -> (-167.2858, -7.8) centre (-167.2858, -6.8) ccw
  arc A117 (-167.2858, 0.2) -> (-167.9929, -0.0929) centre (-167.2858, -0.8) ccw
  line L294 (-167.9929, -7.5071) -> (-170.9, -4.6)
  line L295 (-167.9929, -0.0929) -> (-170.9, -3)
  line L296 (-170.9, -3.8) -> (-170.9, -4.6)
  line L297 (-170.9, -3.8) -> (-170.9, -3)
  line L298 (-167.2858, 0.2) -> (-124.5142, 0.2)
  line L299 (-124.5142, -7.8) -> (-167.2858, -7.8)
  arc A118 (-123.8071, -0.0929) -> (-124.5142, 0.2) centre (-124.5142, -0.8) ccw
  line L300 (-123.8071, -0.0929) -> (-120.9, -3)
  line L301 (-120.9, -3.8) -> (-120.9, -3)
  line L302 (-120.9, -3.8) -> (-120.9, -4.6)
  arc A119 (-124.5142, -7.8) -> (-123.8071, -7.5071) centre (-124.5142, -6.8) ccw
  line L303 (-123.8071, -7.5071) -> (-120.9, -4.6)
  arc A120 (-169.0929, 1.0071) -> (-168.8, 1.7142) centre (-169.8, 1.7142) ccw
  arc A121 (-176.8, 1.7142) -> (-176.5071, 1.0071) centre (-175.8, 1.7142) ccw
  line L304 (-169.0929, 1.0071) -> (-172, -1.9)
  line L305 (-176.5071, 1.0071) -> (-173.6, -1.9)
  line L306 (-172.8, -1.9) -> (-172, -1.9)
  line L307 (-172.8, -1.9) -> (-173.6, -1.9)
  line L308 (-176.8, 1.7142) -> (-176.8, 44.4858)
  line L309 (-168.8, 44.4858) -> (-168.8, 1.7142)
  arc A122 (-176.5071, 45.1929) -> (-176.8, 44.4858) centre (-175.8, 44.4858) ccw
  line L310 (-176.5071, 45.1929) -> (-173.6, 48.1)
  line L311 (-172.8, 48.1) -> (-173.6, 48.1)
  line L312 (-172.8, 48.1) -> (-172, 48.1)
  arc A123 (-168.8, 44.4858) -> (-169.0929, 45.1929) centre (-169.8, 44.4858) ccw
  line L313 (-169.0929, 45.1929) -> (-172, 48.1)
  arc A124 (-169.0929, -52.7929) -> (-168.8, -52.0858) centre (-169.8, -52.0858) ccw
  arc A125 (-176.8, -52.0858) -> (-176.5071, -52.7929) centre (-175.8, -52.0858) ccw
  line L314 (-169.0929, -52.7929) -> (-172, -55.7)
  line L315 (-176.5071, -52.7929) -> (-173.6, -55.7)
  line L316 (-172.8, -55.7) -> (-172, -55.7)
  line L317 (-172.8, -55.7) -> (-173.6, -55.7)
  line L318 (-176.8, -52.0858) -> (-176.8, -9.3142)
  line L319 (-168.8, -9.3142) -> (-168.8, -52.0858)
  arc A126 (-176.5071, -8.6071) -> (-176.8, -9.3142) centre (-175.8, -9.3142) ccw
  line L320 (-176.5071, -8.6071) -> (-173.6, -5.7)
  line L321 (-172.8, -5.7) -> (-173.6, -5.7)
  line L322 (-172.8, -5.7) -> (-172, -5.7)
  arc A127 (-168.8, -9.3142) -> (-169.0929, -8.6071) centre (-169.8, -9.3142) ccw
  line L323 (-169.0929, -8.6071) -> (-172, -5.7)
  arc A128 (-115.2929, 1.0071) -> (-115, 1.7142) centre (-116, 1.7142) ccw
  arc A129 (-123, 1.7142) -> (-122.7071, 1.0071) centre (-122, 1.7142) ccw
  line L324 (-115.2929, 1.0071) -> (-118.2, -1.9)
  line L325 (-122.7071, 1.0071) -> (-119.8, -1.9)
  line L326 (-119, -1.9) -> (-118.2, -1.9)
  line L327 (-119, -1.9) -> (-119.8, -1.9)
  line L328 (-123, 1.7142) -> (-123, 44.4858)
  line L329 (-115, 44.4858) -> (-115, 1.7142)
  arc A130 (-122.7071, 45.1929) -> (-123, 44.4858) centre (-122, 44.4858) ccw
  line L330 (-122.7071, 45.1929) -> (-119.8, 48.1)
  line L331 (-119, 48.1) -> (-119.8, 48.1)
  line L332 (-119, 48.1) -> (-118.2, 48.1)
  arc A131 (-115, 44.4858) -> (-115.2929, 45.1929) centre (-116, 44.4858) ccw
  line L333 (-115.2929, 45.1929) -> (-118.2, 48.1)
  arc A132 (-115.2929, -52.7929) -> (-115, -52.0858) centre (-116, -52.0858) ccw
  arc A133 (-123, -52.0858) -> (-122.7071, -52.7929) centre (-122, -52.0858) ccw
  line L334 (-115.2929, -52.7929) -> (-118.2, -55.7)
  line L335 (-122.7071, -52.7929) -> (-119.8, -55.7)
  line L336 (-119, -55.7) -> (-118.2, -55.7)
  line L337 (-119, -55.7) -> (-119.8, -55.7)
  line L338 (-123, -52.0858) -> (-123, -9.3142)
  line L339 (-115, -9.3142) -> (-115, -52.0858)
  arc A134 (-122.7071, -8.6071) -> (-123, -9.3142) centre (-122, -9.3142) ccw
  line L340 (-122.7071, -8.6071) -> (-119.8, -5.7)
  line L341 (-119, -5.7) -> (-119.8, -5.7)
  line L342 (-119, -5.7) -> (-118.2, -5.7)
  arc A135 (-115, -9.3142) -> (-115.2929, -8.6071) centre (-116, -9.3142) ccw
  line L343 (-115.2929, -8.6071) -> (-118.2, -5.7)
  arc A136 (-167.9929, -61.3071) -> (-167.2858, -61.6) centre (-167.2858, -60.6) ccw
  arc A137 (-167.2858, -53.6) -> (-167.9929, -53.8929) centre (-167.2858, -54.6) ccw
  line L344 (-167.9929, -61.3071) -> (-170.9, -58.4)
  line L345 (-167.9929, -53.8929) -> (-170.9, -56.8)
  line L346 (-170.9, -57.6) -> (-170.9, -58.4)
  line L347 (-170.9, -57.6) -> (-170.9, -56.8)
  line L348 (-167.2858, -53.6) -> (-124.5142, -53.6)
  line L349 (-124.5142, -61.6) -> (-167.2858, -61.6)
  arc A138 (-123.8071, -53.8929) -> (-124.5142, -53.6) centre (-124.5142, -54.6) ccw
  line L350 (-123.8071, -53.8929) -> (-120.9, -56.8)
  line L351 (-120.9, -57.6) -> (-120.9, -56.8)
  line L352 (-120.9, -57.6) -> (-120.9, -58.4)
  arc A139 (-124.5142, -61.6) -> (-123.8071, -61.3071) centre (-124.5142, -60.6) ccw
  line L353 (-123.8071, -61.3071) -> (-120.9, -58.4)
  arc A140 (-285.0929, 27.2929) -> (-284.3858, 27) centre (-284.3858, 28) ccw
  arc A141 (-284.3858, 35) -> (-285.0929, 34.7071) centre (-284.3858, 34) ccw
  line L354 (-285.0929, 27.2929) -> (-288, 30.2)
  line L355 (-285.0929, 34.7071) -> (-288, 31.8)
  line L356 (-288, 31) -> (-288, 30.2)
  line L357 (-288, 31) -> (-288, 31.8)
  line L358 (-284.3858, 35) -> (-241.6142, 35)
  line L359 (-241.6142, 27) -> (-284.3858, 27)
  arc A142 (-240.9071, 34.7071) -> (-241.6142, 35) centre (-241.6142, 34) ccw
  line L360 (-240.9071, 34.7071) -> (-238, 31.8)
  line L361 (-238, 31) -> (-238, 31.8)
  line L362 (-238, 31) -> (-238, 30.2)
  arc A143 (-241.6142, 27) -> (-240.9071, 27.2929) centre (-241.6142, 28) ccw
  line L363 (-240.9071, 27.2929) -> (-238, 30.2)
  arc A144 (216.0071, 46.2929) -> (216.7142, 46) centre (216.7142, 47) ccw
  arc A145 (216.7142, 54) -> (216.0071, 53.7071) centre (216.7142, 53) ccw
  line L364 (216.0071, 46.2929) -> (213.1, 49.2)
  line L365 (216.0071, 53.7071) -> (213.1, 50.8)
  line L366 (213.1, 50) -> (213.1, 49.2)
  line L367 (213.1, 50) -> (213.1, 50.8)
  line L368 (216.7142, 54) -> (259.4858, 54)
  line L369 (259.4858, 46) -> (216.7142, 46)
  arc A146 (260.1929, 53.7071) -> (259.4858, 54) centre (259.4858, 53) ccw
  line L370 (260.1929, 53.7071) -> (263.1, 50.8)
  line L371 (263.1, 50) -> (263.1, 50.8)
  line L372 (263.1, 50) -> (263.1, 49.2)
  arc A147 (259.4858, 46) -> (260.1929, 46.2929) centre (259.4858, 47) ccw
  line L373 (260.1929, 46.2929) -> (263.1, 49.2)
  arc A148 (216.0071, -7.5071) -> (216.7142, -7.8) centre (216.7142, -6.8) ccw
  arc A149 (216.7142, 0.2) -> (216.0071, -0.0929) centre (216.7142, -0.8) ccw
  line L374 (216.0071, -7.5071) -> (213.1, -4.6)
  line L375 (216.0071, -0.0929) -> (213.1, -3)
  line L376 (213.1, -3.8) -> (213.1, -4.6)
  line L377 (213.1, -3.8) -> (213.1, -3)
  line L378 (216.7142, 0.2) -> (259.4858, 0.2)
  line L379 (259.4858, -7.8) -> (216.7142, -7.8)
  arc A150 (260.1929, -0.0929) -> (259.4858, 0.2) centre (259.4858, -0.8) ccw
  line L380 (260.1929, -0.0929) -> (263.1, -3)
  line L381 (263.1, -3.8) -> (263.1, -3)
  line L382 (263.1, -3.8) -> (263.1, -4.6)
  arc A151 (259.4858, -7.8) -> (260.1929, -7.5071) centre (259.4858, -6.8) ccw
  line L383 (260.1929, -7.5071) -> (263.1, -4.6)
  arc A152 (214.9071, 1.0071) -> (215.2, 1.7142) centre (214.2, 1.7142) ccw
  arc A153 (207.2, 1.7142) -> (207.4929, 1.0071) centre (208.2, 1.7142) ccw
  line L384 (214.9071, 1.0071) -> (212, -1.9)
  line L385 (207.4929, 1.0071) -> (210.4, -1.9)
  line L386 (211.2, -1.9) -> (212, -1.9)
  line L387 (211.2, -1.9) -> (210.4, -1.9)
  line L388 (207.2, 1.7142) -> (207.2, 44.4858)
  line L389 (215.2, 44.4858) -> (215.2, 1.7142)
  arc A154 (207.4929, 45.1929) -> (207.2, 44.4858) centre (208.2, 44.4858) ccw
  line L390 (207.4929, 45.1929) -> (210.4, 48.1)
  line L391 (211.2, 48.1) -> (210.4, 48.1)
  line L392 (211.2, 48.1) -> (212, 48.1)
  arc A155 (215.2, 44.4858) -> (214.9071, 45.1929) centre (214.2, 44.4858) ccw
  line L393 (214.9071, 45.1929) -> (212, 48.1)
  arc A156 (214.9071, -52.7929) -> (215.2, -52.0858) centre (214.2, -52.0858) ccw
  arc A157 (207.2, -52.0858) -> (207.4929, -52.7929) centre (208.2, -52.0858) ccw
  line L394 (214.9071, -52.7929) -> (212, -55.7)
  line L395 (207.4929, -52.7929) -> (210.4, -55.7)
  line L396 (211.2, -55.7) -> (212, -55.7)
  line L397 (211.2, -55.7) -> (210.4, -55.7)
  line L398 (207.2, -52.0858) -> (207.2, -9.3142)
  line L399 (215.2, -9.3142) -> (215.2, -52.0858)
  arc A158 (207.4929, -8.6071) -> (207.2, -9.3142) centre (208.2, -9.3142) ccw
  line L400 (207.4929, -8.6071) -> (210.4, -5.7)
  line L401 (211.2, -5.7) -> (210.4, -5.7)
  line L402 (211.2, -5.7) -> (212, -5.7)
  arc A159 (215.2, -9.3142) -> (214.9071, -8.6071) centre (214.2, -9.3142) ccw
  line L403 (214.9071, -8.6071) -> (212, -5.7)
  arc A160 (268.7071, 1.0071) -> (269, 1.7142) centre (268, 1.7142) ccw
  arc A161 (261, 1.7142) -> (261.2929, 1.0071) centre (262, 1.7142) ccw
  line L404 (268.7071, 1.0071) -> (265.8, -1.9)
  line L405 (261.2929, 1.0071) -> (264.2, -1.9)
  line L406 (265, -1.9) -> (265.8, -1.9)
  line L407 (265, -1.9) -> (264.2, -1.9)
  line L408 (261, 1.7142) -> (261, 44.4858)
  line L409 (269, 44.4858) -> (269, 1.7142)
  arc A162 (261.2929, 45.1929) -> (261, 44.4858) centre (262, 44.4858) ccw
  line L410 (261.2929, 45.1929) -> (264.2, 48.1)
  line L411 (265, 48.1) -> (264.2, 48.1)
  line L412 (265, 48.1) -> (265.8, 48.1)
  arc A163 (269, 44.4858) -> (268.7071, 45.1929) centre (268, 44.4858) ccw
  line L413 (268.7071, 45.1929) -> (265.8, 48.1)
  arc A164 (268.7071, -52.7929) -> (269, -52.0858) centre (268, -52.0858) ccw
  arc A165 (261, -52.0858) -> (261.2929, -52.7929) centre (262, -52.0858) ccw
  line L414 (268.7071, -52.7929) -> (265.8, -55.7)
  line L415 (261.2929, -52.7929) -> (264.2, -55.7)
  line L416 (265, -55.7) -> (265.8, -55.7)
  line L417 (265, -55.7) -> (264.2, -55.7)
  line L418 (261, -52.0858) -> (261, -9.3142)
  line L419 (269, -9.3142) -> (269, -52.0858)
  arc A166 (261.2929, -8.6071) -> (261, -9.3142) centre (262, -9.3142) ccw
  line L420 (261.2929, -8.6071) -> (264.2, -5.7)
  line L421 (265, -5.7) -> (264.2, -5.7)
  line L422 (265, -5.7) -> (265.8, -5.7)
  arc A167 (269, -9.3142) -> (268.7071, -8.6071) centre (268, -9.3142) ccw
  line L423 (268.7071, -8.6071) -> (265.8, -5.7)
  arc A168 (216.0071, -61.3071) -> (216.7142, -61.6) centre (216.7142, -60.6) ccw
  arc A169 (216.7142, -53.6) -> (216.0071, -53.8929) centre (216.7142, -54.6) ccw
  line L424 (216.0071, -61.3071) -> (213.1, -58.4)
  line L425 (216.0071, -53.8929) -> (213.1, -56.8)
  line L426 (213.1, -57.6) -> (213.1, -58.4)
  line L427 (213.1, -57.6) -> (213.1, -56.8)
  line L428 (216.7142, -53.6) -> (259.4858, -53.6)
  line L429 (259.4858, -61.6) -> (216.7142, -61.6)
  arc A170 (260.1929, -53.8929) -> (259.4858, -53.6) centre (259.4858, -54.6) ccw
  line L430 (260.1929, -53.8929) -> (263.1, -56.8)
  line L431 (263.1, -57.6) -> (263.1, -56.8)
  line L432 (263.1, -57.6) -> (263.1, -58.4)
  arc A171 (259.4858, -61.6) -> (260.1929, -61.3071) centre (259.4858, -60.6) ccw
  line L433 (260.1929, -61.3071) -> (263.1, -58.4)
  line L434 (-262.2, 25.9) -> (-263.8, 25.9)
  line L435 (-263.8, 25.9) -> (-267, 22.7)
  line L436 (-267, 22.7) -> (-271.0621, -34.3)
  line L437 (-263.0621, -34.3) -> (-259, 22.7)
  line L438 (-259, 22.7) -> (-262.2, 25.9)
  line L439 (-271.0621, -34.3) -> (-267.8621, -37.5)
  line L440 (-267.8621, -37.5) -> (-266.2621, -37.5)
  line L441 (-266.2621, -37.5) -> (-263.0621, -34.3)
  line L442 (-217, 20.5) -> (-219.9071, 17.5929)
  line L443 (-220.2, 16.8858) -> (-220.2, -0.3)
  line L444 (-237.3858, -0.3) -> (-220.2, -0.3)
  line L445 (-238.0929, -0.5929) -> (-241, -3.5)
  line L446 (-241, -3.5) -> (-241, -5.1)
  line L447 (-237.3858, -8.3) -> (-220.2, -8.3)
  line L448 (-220.2, -8.3) -> (-220.2, -25.4858)
  line L449 (-217, -29.1) -> (-215.4, -29.1)
  line L450 (-215.4, -29.1) -> (-212.4929, -26.1929)
  line L451 (-212.2, -25.4858) -> (-212.2, -8.3)
  line L452 (-195.0142, -0.3) -> (-212.2, -0.3)
  line L453 (-195.0142, -8.3) -> (-212.2, -8.3)
  line L454 (-194.3071, -0.5929) -> (-191.4, -3.5)
  line L455 (-191.4, -3.5) -> (-191.4, -5.1)
  line L456 (-238.0929, -8.0071) -> (-241, -5.1)
  line L457 (-219.9071, -26.1929) -> (-217, -29.1)
  line L458 (-194.3071, -8.0071) -> (-191.4, -5.1)
  line L459 (-212.2, -0.3) -> (-212.2, 16.8858)
  line L460 (-212.4929, 17.5929) -> (-215.4, 20.5)
  line L461 (-215.4, 20.5) -> (-217, 20.5)
  arc A172 (-219.9071, 17.5929) -> (-220.2, 16.8858) centre (-219.2, 16.8858) ccw
  arc A173 (-212.2, 16.8858) -> (-212.4929, 17.5929) centre (-213.2, 16.8858) ccw
  arc A174 (-194.3071, -0.5929) -> (-195.0142, -0.3) centre (-195.0142, -1.3) ccw
  arc A175 (-195.0142, -8.3) -> (-194.3071, -8.0071) centre (-195.0142, -7.3) ccw
  arc A176 (-220.2, -25.4858) -> (-219.9071, -26.1929) centre (-219.2, -25.4858) ccw
  arc A177 (-212.4929, -26.1929) -> (-212.2, -25.4858) centre (-213.2, -25.4858) ccw
  arc A178 (-238.0929, -8.0071) -> (-237.3858, -8.3) centre (-237.3858, -7.3) ccw
  arc A179 (-237.3858, -0.3) -> (-238.0929, -0.5929) centre (-237.3858, -1.3) ccw
  line L462 (-34.2, 15) -> (-32.2, 15)
  line L463 (-32.2, 15) -> (-29, 11.8)
  line L464 (-29, 11.8) -> (-29, 9.8)
  line L465 (-29, 9.8) -> (-32.2, 6.6)
  line L466 (-32.2, 6.6) -> (-34.2, 6.6)
  line L467 (-34.2, 6.6) -> (-37.4, 9.8)
  line L468 (-37.4, 9.8) -> (-37.4, 11.8)
  line L469 (-37.4, 11.8) -> (-34.2, 15)
  line L470 (-34.2, -14.4) -> (-32.2, -14.4)
  line L471 (-32.2, -14.4) -> (-29, -17.6)
  line L472 (-29, -17.6) -> (-29, -19.6)
  line L473 (-29, -19.6) -> (-32.2, -22.8)
  line L474 (-32.2, -22.8) -> (-34.2, -22.8)
  line L475 (-34.2, -22.8) -> (-37.4, -19.6)
  line L476 (-37.4, -19.6) -> (-37.4, -17.6)
  line L477 (-37.4, -17.6) -> (-34.2, -14.4)
  line L478 (121.9, 15) -> (123.9, 15)
  line L479 (123.9, 15) -> (127.1, 11.8)
  line L480 (127.1, 11.8) -> (127.1, 9.8)
  line L481 (127.1, 9.8) -> (123.9, 6.6)
  line L482 (123.9, 6.6) -> (121.9, 6.6)
  line L483 (121.9, 6.6) -> (118.7, 9.8)
  line L484 (118.7, 9.8) -> (118.7, 11.8)
  line L485 (118.7, 11.8) -> (121.9, 15)
  line L486 (121.9, -14.4) -> (123.9, -14.4)
  line L487 (123.9, -14.4) -> (127.1, -17.6)
  line L488 (127.1, -17.6) -> (127.1, -19.6)
  line L489 (127.1, -19.6) -> (123.9, -22.8)
  line L490 (123.9, -22.8) -> (121.9, -22.8)
  line L491 (121.9, -22.8) -> (118.7, -19.6)
  line L492 (118.7, -19.6) -> (118.7, -17.6)
  line L493 (118.7, -17.6) -> (121.9, -14.4)
  point P0 (0, 0)
extrude "Extrusion2" cut sketch "Sketch4" against normal blind 3
body "Solid1"
